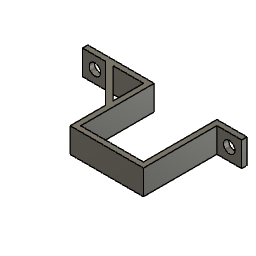
MotorBracket (Autodesk Fusion 360 design; units mm, degrees)
Autodesk Fusion 360 part; units mm, degrees
sketch "Sketch1" plane through (0, 0, 0) normal (0, 1, 0) x (1, 0, 0)
  line L0 (0, 0) -> (19, 0)
  line L1 (19, 0) -> (19, 22.5)
  line L2 (19, 22.5) -> (0, 22.5)
  line L3 (0, 22.5) -> (0, 0)
  dimension "d1" = 19
  dimension "d2" = 22.5
  constraint horizontal L0
  constraint vertical L1
  constraint horizontal L2
  constraint vertical L3
  constraint coincident L0.start L3.end
  measures "d1" distance of L0.start L0.end
  measures "d2" distance of L0.end L1.end
extrude "Extrude1" add sketch "Sketch1" along normal blind 20 makes body 1
sketch "Sketch2" plane through (0, 0, 0) normal (0, 0, 1) x (1, 0, 0)
  line L0 (0, 0) -> (19, 0)
  line L1 (19, 0) -> (19, 20)
  line L2 (19, 20) -> (0, 20)
  line L3 (0, 20) -> (0, 0)
  line L4 (20.6, 7.5) -> (-1.6, 7.5)
  line L5 (-1.6, 7.5) -> (-1.6, 0)
  line L6 (-1.6, 0) -> (20.6, 0)
  line L7 (20.6, 0) -> (20.6, 7.5)
  line L8 (19, 7.5) -> (19, 0)
  line L9 (0, 7.5) -> (0, 0)
  dimension "d5" = 1.6
  dimension "d6" = 1.6
  dimension "d7" = 7.5
  constraint horizontal L4
  constraint vertical L5
  constraint horizontal L6
  constraint vertical L7
  constraint coincident L1 L8.start
  constraint coincident L4 L8.start
  constraint coincident L4 L9.start
  constraint coincident L3 L9.start
  constraint coincident L6 L0.end
  constraint coincident L6 L0.start
  constraint coincident L0.start L6
  measures "d5" distance of L1 L7
  measures "d6" distance of L3 L5
  measures "d7" distance of L4.start L6.end
extrude "Extrude2" add sketch "Sketch2" against normal blind 22.25 separate body contours L3 L4 L5 L6 L9 | L1 L4 L6 L7 L8 makes body 2 at (19, 2.5, -7.4167) makes body 3 at (-1.6, 5, -7.4167)
extrude "Extrude3" add sketch "Sketch2" along normal blind 1.6 separate body contours L0 L1 L3 L4 L6 L8 L9 | L3 L4 L5 L6 L9 | L1 L4 L6 L7 L8 makes body 4
combine "Combine1" operation add target body 2 tool bodies 4 3
sketch "Sketch3" plane through (0, 0, -22.25) normal (0, 0, -1) x (-1, 0, 0)
  line L0 (1.6, 0) -> (1.6, 7.5)
  line L1 (1.6, 7.5) -> (0, 7.5)
  line L2 (0, 7.5) -> (0, 0)
  line L3 (0, 0) -> (1.6, 0)
  line L4 (1.6, 0) -> (20.1, 0)
  line L5 (20.1, 0) -> (20.1, 7.5)
  line L6 (20.1, 7.5) -> (1.6, 7.5)
  line L7 (1.6, 7.5) -> (1.6, 0)
  line L8 (-20.6, 0) -> (-28.1, 0)
  line L9 (-28.1, 0) -> (-28.1, 7.5)
  line L10 (-28.1, 7.5) -> (-20.6, 7.5)
  line L11 (-20.6, 7.5) -> (-20.6, 0)
  line L12 (-19, 7.5) -> (-20.6, 7.5)
  circle A0 centre (-24.35, 3.75) radius 1.75
  circle A1 centre (16.35, 3.75) radius 1.75
  point P0 (-20.6, 0)
  dimension "d13" = 7.5
  dimension "d16" = 3.5
  dimension "d17" = 3.75
  dimension "d18" = 3.75
  dimension "d19" = 3.75
  dimension "d20" = 3.75
  dimension "d29" = 40.7
  constraint horizontal L4
  constraint vertical L5
  constraint horizontal L6
  constraint vertical L7
  constraint coincident L0.start L3.end
  constraint collinear L1 L6
  constraint horizontal L8
  constraint vertical L9
  constraint horizontal L10
  constraint vertical L11
  constraint coincident P0 L8.start
  constraint collinear L10 L12
  constraint equal A0 A1
  measures "d13" distance of P0 L8.end
  measures "d16" diameter of A1
  measures "d17" distance of L10 A0.centre
  measures "d18" distance of L9 A0.centre
  measures "d19" distance of L6 A1.centre
  measures "d20" distance of L5 A1.centre
  measures "d29" distance of A0.centre A1.centre
extrude "Extrude4" add sketch "Sketch3" against normal blind 1.6 contours L0 L4 L5 L6 L7 | L8 L9 L10 L11 bodies 2
chamfer "Chamfer1" distance 11.5 angle 45 1 edges at (-1.6, 3.75, -20.65) on bodies 2
sketch "Sketch6" plane through (0, 7.5, 0) normal (0, 1, 0) x (-1, 0, 0)
  line L0 (-28.1, -22.25) -> (-19, -22.25)
  line L1 (-19, -22.25) -> (-19, 0)
  line L2 (-19, 0) -> (0, 0)
  line L3 (0, 0) -> (0, -22.25)
  line L4 (0, -22.25) -> (20.1, -22.25)
  line L5 (20.1, -22.25) -> (20.1, -20.65)
  line L6 (20.1, -20.65) -> (13.1, -20.65)
  line L7 (13.1, -20.65) -> (1.6, -9.15)
  line L8 (1.6, -9.15) -> (1.6, 1.6)
  line L9 (1.6, 1.6) -> (-20.6, 1.6)
  line L10 (-20.6, 1.6) -> (-20.6, -20.65)
  line L11 (-20.6, -20.65) -> (-28.1, -20.65)
  line L12 (-28.1, -20.65) -> (-28.1, -22.25)
  line L13 (1.6, -11.4127) -> (10.8373, -20.65)
  line L14 (10.8373, -20.65) -> (1.6, -20.65)
  line L15 (1.6, -20.65) -> (1.6, -11.4127)
  dimension "d23" = 1.6
  dimension "d24" = 1.6
  dimension "d25" = 1.6
  constraint parallel L7 L13
  constraint horizontal L14
  constraint perpendicular L14 L15
  measures "d23" distance of L4 L14
  measures "d24" distance of L7 L13
  measures "d25" distance of L3 L15
extrude "Extrude5" cut sketch "Sketch6" against normal blind 11 contours L13 L14 L15 bodies 2
hidden bodies 1
equation "d17 = ( 7.5 / 2 ) * 1 mm"
equation "d18 = ( 7.5 / 2 ) * 1 mm"
equation "d19 = ( 7.5 / 2 ) * 1 mm"
equation "d20 = ( 7.5 / 2 ) * 1 mm"
